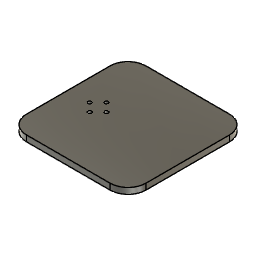
Arm Assembly v5 (Autodesk Fusion 360 archive; units mm, degrees)
design "Base"
Autodesk Fusion 360 part; units mm, degrees
sketch "Sketch1" plane through (0, 0, 0) normal (0, 0, 1) x (1, 0, 0)
  circle A0 centre (0, 0) radius 5
  circle A1 centre (0, 0) radius 10
  circle A2 centre (-7, 0) radius 1.5
  circle A3 centre (0, -7) radius 1.5
  circle A4 centre (0, 0) radius 7 construction
  circle A5 centre (7, 0) radius 1.5
  circle A6 centre (0, 7) radius 1.5
  line L0 (-10, 50) -> (60, 50)
  line L1 (75, 35) -> (75, -35)
  line L2 (60, -50) -> (-10, -50)
  line L3 (-25, -35) -> (-25, 35)
  arc A7 (-10, 50) -> (-25, 35) centre (-10, 35) ccw
  arc A8 (75, 35) -> (60, 50) centre (60, 35) ccw
  arc A9 (-25, -35) -> (-10, -50) centre (-10, -35) ccw
  arc A10 (60, -50) -> (75, -35) centre (60, -35) ccw
  point P0 (0, -9.2368)
  point P1 (-25, 50)
  point P2 (75, 50)
  point P3 (-25, -50)
  dimension "d2" = 360
  dimension "d3" = 14
  dimension "d4" = 3
  dimension "d5" = 20
  dimension "d6" = 10
  dimension "d11" = 100
  dimension "d12" = 100
  dimension "d13" = 25
  dimension "d15" = 50
  dimension "d19" = 15
  dimension "d20" = 15
  constraint coincident A6.centre A4
  constraint vertical A6.centre A0.centre
  constraint coincident A0.centre A1.centre
  constraint concentric A1 A4
  constraint concentric A0 A4
  constraint horizontal L0
  constraint vertical L1
  constraint horizontal L2
  constraint vertical L3
  constraint coincident P1 L0
  constraint coincident P1 L3
  constraint tangent L0 A7
  constraint tangent L3 A7
  constraint coincident P2 L0
  constraint coincident P2 L1
  constraint tangent L0 A8
  constraint tangent L1 A8
  constraint equal A7 A8
  constraint coincident P3 L2
  constraint coincident P3 L3
  constraint tangent L2 A9
  constraint tangent L3 A9
  constraint tangent L1 A10
  constraint tangent L2 A10
  constraint equal A9 A10
  measures "d3" diameter of A4
  measures "d4" diameter of A6
  measures "d5" diameter of A1
  measures "d6" diameter of A0
  measures "d11" distance of P1 P2
  measures "d12" distance of P1 P3
  measures "d13" distance of A0.centre L3
  measures "d15" distance of A0.centre L0
  measures "d19" radius of A7
  measures "d20" radius of A9
extrude "Extrude1" add sketch "Sketch1" along normal blind 5 contours A0 | A1 | L0 L1 L2 L3 A7 A8 A9 A10
equation "base_length = 100 mm"
equation "base_height = 5 mm"
equation "base_horizontal = 25 mm"
equation "base_vertical = base_length / 2"
equation "d11 = base_length"
equation "d12 = base_length"
equation "d13 = base_horizontal"
equation "d15 = base_vertical"
equation "d16 = base_height"
equation "base_filet = 15 mm"
equation "d19 = base_filet"
equation "d20 = base_filet"
